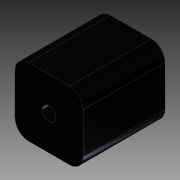
# Autodesk Inventor part: block
Saved by Autodesk Inventor 2015 (Build 190159000, 159)
## iProperties
Created: 2015-12-03
Part Number: block
Material: Generic
Document SubType Name: Modeling
Designer: david
Density: 1 g/cm^3
Appearance: Black
Mass: 0.0175171 g
Surface Area: 0.438153 cm^2
Volume: 0.0175171 cm^3
Author: david
Autodesk Inventor part; units mm, degrees
ref_plane "YZ Plane" through (0, 0, 0) normal (1, 0, 0) x (0, 1, 0)
ref_plane "XZ Plane" through (0, 0, 0) normal (0, 1, 0) x (-1, 0, 0)
ref_plane "XY Plane" through (0, 0, 0) normal (0, 0, 1) x (1, 0, 0)
sketch "Sketch1" plane through (0, 0, 0) normal (0, 1, 0) x (-1, 0, 0)
  line L0 (-1.25, 1.25) -> (1.25, 1.25)
  line L1 (1.25, 1.25) -> (1.25, -1.25)
  line L2 (1.25, -1.25) -> (-1.25, -1.25)
  line L3 (-1.25, -1.25) -> (-1.25, 1.25)
  line L4 (-1.25, 1.25) -> (1.25, -1.25) construction
  line L5 (1.25, 1.25) -> (-1.25, -1.25) construction
  point P0 (0, 0)
  dimension "d0" = 2.5
  dimension "d1" = 2.5
  constraints: 12 end point, 2 midpoint, 2 parallel, 1 horizontal, 1 perpendicular
  measures "d0" distance of L1.end L2.end
  measures "d1" distance of L0.end L1.end
extrude "Extrusion1" add sketch "Sketch1" along normal blind 3
fillet "Fillet1" radius 0.5 4 edges at (-1.25, 1.5, 1.25) (1.25, 1.5, 1.25) (1.25, 1.5, -1.25) (-1.25, 1.5, -1.25)
sketch "Sketch2" plane through (0, 3, 0) normal (0, 1, 0) x (1, 0, 0)
  circle A0 centre (0, 0) radius 0.25
  dimension "d5" = 0.5
  constraints: 1 centre point, 1 coincident
  measures "d5" diameter of A0
extrude "Extrusion2" cut sketch "Sketch2" against normal blind 3
body "Solid1"
